Autodesk Inventor part; units mm, degrees
(part 2 of 2)
sketch "Эскиз18" plane through (0, 0, 0) normal (0, 0, -1) x (-1, 0, 0)
  line L0 (-71.0437, 196.2632) -> (-89.8727, 218.3448) projected
  arc A0 (-86.829, 224.9401) -> (-89.8727, 218.3448) centre (-86.829, 220.9401) ccw projected
  line L1 (-86.829, 224.9401) -> (-49.171, 224.9401) projected
  arc A1 (-46.1273, 218.3448) -> (-49.171, 224.9401) centre (-49.171, 220.9401) ccw projected
  line L2 (-46.1273, 218.3448) -> (-64.9563, 196.2632) projected
  arc A2 (-71.0437, 196.2632) -> (-64.9563, 196.2632) centre (-68, 198.8586) ccw projected
  line L3 (-53.9492, 66.9978) -> (-53.9492, 50.0917) projected
  arc A3 (-57.1492, 50.0917) -> (-53.9492, 50.0917) centre (-55.5492, 50.0917) ccw projected
  line L4 (-57.1492, 50.0917) -> (-57.1492, 66.9978) projected
  arc A4 (-53.9492, 66.9978) -> (-57.1492, 66.9978) centre (-55.5492, 66.9978) ccw projected
  line L5 (-23.75, 263.345) -> (-23.75, 243.345) projected
  arc A5 (-50.25, 243.345) -> (-23.75, 243.345) centre (-37, 243.345) ccw projected
  line L6 (-50.25, 243.345) -> (-50.25, 263.345) projected
  arc A6 (-23.75, 263.345) -> (-50.25, 263.345) centre (-37, 263.345) ccw projected
  line L7 (-54.45, 263.345) -> (-54.45, 243.345) projected
  arc A7 (-58.75, 243.345) -> (-54.45, 243.345) centre (-56.6, 243.345) ccw projected
  line L8 (-58.75, 243.345) -> (-58.75, 263.345) projected
  arc A8 (-54.45, 263.345) -> (-58.75, 263.345) centre (-56.6, 263.345) ccw projected
  line L9 (-19.55, 243.345) -> (-19.55, 263.345) projected
  arc A9 (-15.25, 263.345) -> (-19.55, 263.345) centre (-17.4, 263.345) ccw projected
  line L10 (-15.25, 263.345) -> (-15.25, 243.345) projected
  arc A10 (-19.55, 243.345) -> (-15.25, 243.345) centre (-17.4, 243.345) ccw projected
  line L11 (-59.5472, 66.9978) -> (-59.5472, 50.6) projected
  arc A11 (-83.5472, 50.6) -> (-59.5472, 50.6) centre (-71.5472, 50.6) ccw projected
  line L12 (-83.5472, 50.6) -> (-83.5472, 66.9978) projected
  arc A12 (-59.5472, 66.9978) -> (-83.5472, 66.9978) centre (-71.5472, 66.9978) ccw projected
  line L13 (-89.1248, 51.1083) -> (-89.1248, 58.7989) projected
  arc A13 (-89.1248, 59.3072) -> (-89.1248, 58.7989) centre (-87.5451, 59.053) ccw projected
  line L14 (-89.1248, 59.3072) -> (-89.1248, 66.9978) projected
  arc A14 (-85.9655, 66.9978) -> (-89.1248, 66.9978) centre (-87.5451, 66.9978) ccw projected
  line L15 (-85.9655, 66.9978) -> (-85.9655, 59.3072) projected
  arc A15 (-85.9655, 58.7989) -> (-85.9655, 59.3072) centre (-87.5451, 59.053) ccw projected
  line L16 (-85.9655, 58.7989) -> (-85.9655, 51.1083) projected
  arc A16 (-89.1248, 51.1083) -> (-85.9655, 51.1083) centre (-87.5451, 51.1083) ccw projected
  line L17 (-26.8046, 136.6761) -> (-52.0917, 166.3314) projected
  arc A17 (-52.0917, 172.8198) -> (-52.0917, 166.3314) centre (-48.2871, 169.5756) ccw projected
  line L18 (-52.0917, 172.8198) -> (-26.8046, 202.4751) projected
  arc A18 (-18, 199.2309) -> (-26.8046, 202.4751) centre (-23, 199.2309) ccw projected
  line L19 (-18, 199.2309) -> (-18, 139.9204) projected
  arc A19 (-26.8046, 136.6761) -> (-18, 139.9204) centre (-23, 139.9204) ccw projected
  line L20 (-109.1954, 202.4751) -> (-83.9083, 172.8198) projected
  arc A20 (-83.9083, 166.3314) -> (-83.9083, 172.8198) centre (-87.7129, 169.5756) ccw projected
  line L21 (-83.9083, 166.3314) -> (-109.1954, 136.6761) projected
  arc A21 (-118, 139.9204) -> (-109.1954, 136.6761) centre (-113, 139.9204) ccw projected
  line L22 (-118, 139.9204) -> (-118, 199.2309) projected
  arc A22 (-109.1954, 202.4751) -> (-118, 199.2309) centre (-113, 199.2309) ccw projected
  line L23 (-99.3012, 117.4553) -> (-71.8046, 149.7017) projected
  arc A23 (-64.1954, 149.7017) -> (-71.8046, 149.7017) centre (-68, 146.4575) ccw projected
  line L24 (-64.1954, 149.7017) -> (-36.6988, 117.4553) projected
  arc A24 (-40.5034, 109.2111) -> (-36.6988, 117.4553) centre (-40.5034, 114.2111) ccw projected
  line L25 (-40.5034, 109.2111) -> (-95.4966, 109.2111) projected
  arc A25 (-99.3012, 117.4553) -> (-95.4966, 109.2111) centre (-95.4966, 114.2111) ccw projected
  arc A26 (-4.2138, 22.4317) -> (0, 27.3695) centre (-5, 27.3695) ccw projected
  line L26 (0, 267.9415) -> (0, 27.3695) projected
  arc A27 (0, 267.9415) -> (-13.124, 288.8888) centre (-37, 259.345) ccw projected
  arc A28 (-13.124, 288.8888) -> (-16.2668, 290) centre (-16.2668, 285) ccw projected
  line L27 (-16.2668, 290) -> (-72.7377, 290) projected
  arc A29 (-72.7377, 290) -> (-74.4347, 289.7032) centre (-72.7377, 285) ccw projected
  arc A30 (-74.4347, 289.7032) -> (-150, 221.3595) centre (-28.8449, 163.3493) ccw projected
  line L28 (-150, 62.7066) -> (-150, 221.3595) projected
  arc A31 (-150, 62.7066) -> (-147.5924, 58.4311) centre (-145, 62.7066) ccw projected
  arc A32 (-147.1688, 58.1436) -> (-147.5924, 58.4311) centre (-150.1848, 54.1556) ccw projected
  arc A33 (-147.1688, 58.1436) -> (-4.2138, 22.4317) centre (-33.7733, 208.0855) ccw projected
  circle A34 centre (-27.8653, 29.2915) radius 2.1 projected
  circle A35 centre (-62, 278.7903) radius 2.1 projected
  circle A36 centre (-19, 278.7903) radius 2.1 projected
  circle A37 centre (-46.8597, 40.7124) radius 5.5 projected
  circle A38 centre (-8, 239.9401) radius 2.25 projected
  circle A39 centre (-8, 169.5272) radius 2.25 projected
  circle A40 centre (-8, 99.2111) radius 2.25 projected
  circle A41 centre (-81, 273) radius 5.5 projected
  circle A42 centre (-115, 59.0909) radius 5.5 projected
  circle A43 centre (-94.3579, 89.0409) radius 2.25 projected
  circle A44 centre (-142.3579, 79.1409) radius 2.25 projected
  circle A45 centre (-94.3579, 79.1409) radius 2.25 projected
  circle A46 centre (-142.3579, 89.0409) radius 2.25 projected
  line L29 (-37, 290) -> (-37, 255.5)
  circle A47 centre (-37, 255.5) radius 13.25
  circle A48 centre (-37, 239.745) radius 2.1 projected
  circle A49 centre (-37, 278.945) radius 2.1 projected
  line L30 (-37, 255.5) -> (-56.6, 255.5)
  circle A50 centre (-56.6, 255.5) radius 2.15
  circle A51 centre (-37, 235.9) radius 2.15
  circle A52 centre (-17.4, 255.5) radius 2.15
  circle A53 centre (-37, 275.1) radius 2.15
  line L31 (-71.0437, 196.2632) -> (-89.8727, 218.3448) projected
  arc A54 (-86.829, 224.9401) -> (-89.8727, 218.3448) centre (-86.829, 220.9401) ccw projected
  line L32 (-86.829, 224.9401) -> (-49.171, 224.9401) projected
  arc A55 (-46.1273, 218.3448) -> (-49.171, 224.9401) centre (-49.171, 220.9401) ccw projected
  line L33 (-46.1273, 218.3448) -> (-64.9563, 196.2632) projected
  arc A56 (-71.0437, 196.2632) -> (-64.9563, 196.2632) centre (-68, 198.8586) ccw projected
  line L34 (-53.9492, 66.9978) -> (-53.9492, 50.0917) projected
  arc A57 (-57.1492, 50.0917) -> (-53.9492, 50.0917) centre (-55.5492, 50.0917) ccw projected
  line L35 (-57.1492, 50.0917) -> (-57.1492, 66.9978) projected
  arc A58 (-53.9492, 66.9978) -> (-57.1492, 66.9978) centre (-55.5492, 66.9978) ccw projected
  line L36 (-23.75, 263.345) -> (-23.75, 243.345) projected
  arc A59 (-50.25, 243.345) -> (-23.75, 243.345) centre (-37, 243.345) ccw projected
  line L37 (-50.25, 243.345) -> (-50.25, 263.345) projected
  arc A60 (-23.75, 263.345) -> (-50.25, 263.345) centre (-37, 263.345) ccw projected
  line L38 (-54.45, 263.345) -> (-54.45, 243.345) projected
  arc A61 (-58.75, 243.345) -> (-54.45, 243.345) centre (-56.6, 243.345) ccw projected
  line L39 (-58.75, 243.345) -> (-58.75, 263.345) projected
  arc A62 (-54.45, 263.345) -> (-58.75, 263.345) centre (-56.6, 263.345) ccw projected
  line L40 (-19.55, 243.345) -> (-19.55, 263.345) projected
  arc A63 (-15.25, 263.345) -> (-19.55, 263.345) centre (-17.4, 263.345) ccw projected
  line L41 (-15.25, 263.345) -> (-15.25, 243.345) projected
  arc A64 (-19.55, 243.345) -> (-15.25, 243.345) centre (-17.4, 243.345) ccw projected
  line L42 (-59.5472, 66.9978) -> (-59.5472, 50.6) projected
  arc A65 (-83.5472, 50.6) -> (-59.5472, 50.6) centre (-71.5472, 50.6) ccw projected
  line L43 (-83.5472, 50.6) -> (-83.5472, 66.9978) projected
  arc A66 (-59.5472, 66.9978) -> (-83.5472, 66.9978) centre (-71.5472, 66.9978) ccw projected
  line L44 (-89.1248, 51.1083) -> (-89.1248, 58.7989) projected
  arc A67 (-89.1248, 59.3072) -> (-89.1248, 58.7989) centre (-87.5451, 59.053) ccw projected
  line L45 (-89.1248, 59.3072) -> (-89.1248, 66.9978) projected
  arc A68 (-85.9655, 66.9978) -> (-89.1248, 66.9978) centre (-87.5451, 66.9978) ccw projected
  line L46 (-85.9655, 66.9978) -> (-85.9655, 59.3072) projected
  arc A69 (-85.9655, 58.7989) -> (-85.9655, 59.3072) centre (-87.5451, 59.053) ccw projected
  line L47 (-85.9655, 58.7989) -> (-85.9655, 51.1083) projected
  arc A70 (-89.1248, 51.1083) -> (-85.9655, 51.1083) centre (-87.5451, 51.1083) ccw projected
  line L48 (-26.8046, 136.6761) -> (-52.0917, 166.3314) projected
  arc A71 (-52.0917, 172.8198) -> (-52.0917, 166.3314) centre (-48.2871, 169.5756) ccw projected
  line L49 (-52.0917, 172.8198) -> (-26.8046, 202.4751) projected
  arc A72 (-18, 199.2309) -> (-26.8046, 202.4751) centre (-23, 199.2309) ccw projected
  line L50 (-18, 199.2309) -> (-18, 139.9204) projected
  arc A73 (-26.8046, 136.6761) -> (-18, 139.9204) centre (-23, 139.9204) ccw projected
  line L51 (-109.1954, 202.4751) -> (-83.9083, 172.8198) projected
  arc A74 (-83.9083, 166.3314) -> (-83.9083, 172.8198) centre (-87.7129, 169.5756) ccw projected
  line L52 (-83.9083, 166.3314) -> (-109.1954, 136.6761) projected
  arc A75 (-118, 139.9204) -> (-109.1954, 136.6761) centre (-113, 139.9204) ccw projected
  line L53 (-118, 139.9204) -> (-118, 199.2309) projected
  arc A76 (-109.1954, 202.4751) -> (-118, 199.2309) centre (-113, 199.2309) ccw projected
  line L54 (-99.3012, 117.4553) -> (-71.8046, 149.7017) projected
  arc A77 (-64.1954, 149.7017) -> (-71.8046, 149.7017) centre (-68, 146.4575) ccw projected
  line L55 (-64.1954, 149.7017) -> (-36.6988, 117.4553) projected
  arc A78 (-40.5034, 109.2111) -> (-36.6988, 117.4553) centre (-40.5034, 114.2111) ccw projected
  line L56 (-40.5034, 109.2111) -> (-95.4966, 109.2111) projected
  arc A79 (-99.3012, 117.4553) -> (-95.4966, 109.2111) centre (-95.4966, 114.2111) ccw projected
  arc A80 (-4.2138, 22.4317) -> (0, 27.3695) centre (-5, 27.3695) ccw projected
  line L57 (0, 267.9415) -> (0, 27.3695) projected
  arc A81 (0, 267.9415) -> (-13.124, 288.8888) centre (-37, 259.345) ccw projected
  arc A82 (-13.124, 288.8888) -> (-16.2668, 290) centre (-16.2668, 285) ccw projected
  line L58 (-16.2668, 290) -> (-72.7377, 290) projected
  arc A83 (-72.7377, 290) -> (-74.4347, 289.7032) centre (-72.7377, 285) ccw projected
  arc A84 (-74.4347, 289.7032) -> (-150, 221.3595) centre (-28.8449, 163.3493) ccw projected
  line L59 (-150, 62.7066) -> (-150, 221.3595) projected
  arc A85 (-150, 62.7066) -> (-147.5924, 58.4311) centre (-145, 62.7066) ccw projected
  arc A86 (-147.1688, 58.1436) -> (-147.5924, 58.4311) centre (-150.1848, 54.1556) ccw projected
  arc A87 (-147.1688, 58.1436) -> (-4.2138, 22.4317) centre (-33.7733, 208.0855) ccw projected
  circle A88 centre (-27.8653, 29.2915) radius 2.1 projected
  circle A89 centre (-62, 278.7903) radius 2.1 projected
  circle A90 centre (-19, 278.7903) radius 2.1 projected
  circle A91 centre (-46.8597, 40.7124) radius 5.5 projected
  circle A92 centre (-8, 239.9401) radius 2.25 projected
  circle A93 centre (-8, 169.5272) radius 2.25 projected
  circle A94 centre (-8, 99.2111) radius 2.25 projected
  circle A95 centre (-81, 273) radius 5.5 projected
  circle A96 centre (-115, 59.0909) radius 5.5 projected
  circle A97 centre (-94.3579, 89.0409) radius 2.25 projected
  circle A98 centre (-142.3579, 79.1409) radius 2.25 projected
  circle A99 centre (-94.3579, 79.1409) radius 2.25 projected
  circle A100 centre (-142.3579, 89.0409) radius 2.25 projected
  circle A101 centre (-37, 255.5) radius 198.341
  line L60 (-71.5472, 50.6) -> (-71.5472, 66.9978)
  circle A102 centre (-71.5472, 60.1909) radius 12
  line L61 (-71.5472, 60.1909) -> (-93.4927, 60.1909)
  line L62 (-87.5451, 59.053) -> (-87.5451, 66.9978)
  circle A103 centre (-87.5451, 60.1909) radius 1.6
  circle A104 centre (-71.5472, 44.1929) radius 1.6
  circle A105 centre (-55.5492, 60.1909) radius 1.6
  circle A106 centre (-71.5472, 76.1889) radius 1.6
  line L63 (-40.5034, 229.9401) -> (-95.4966, 229.9401)
  line L64 (-99.3012, 221.6959) -> (-71.8046, 189.4495)
  line L65 (-64.1954, 189.4495) -> (-36.6988, 221.6959)
  arc A107 (-71.8046, 189.4495) -> (-64.1954, 189.4495) centre (-68, 192.6937) ccw
  arc A108 (-95.4966, 229.9401) -> (-99.3012, 221.6959) centre (-95.4966, 224.9401) ccw
  arc A109 (-36.6988, 221.6959) -> (-40.5034, 229.9401) centre (-40.5034, 224.9401) ccw
  point P0 (0, 0)
  point P1 (-15.25, 255.5)
  point P2 (-19.55, 255.5)
  point P3 (-58.75, 255.5)
  point P4 (-54.45, 255.5)
  point P5 (-35.3627, 276.4934)
  point P6 (-38.6373, 276.4934)
  point P7 (-50.25, 255.5)
  point P8 (-23.75, 255.5)
  point P9 (-53.9492, 60.1909)
  point P10 (-57.1492, 60.1909)
  point P11 (-89.1248, 60.445)
  point P12 (-85.9655, 60.445)
  point P13 (-85.9655, 59.9368)
  point P14 (-89.1248, 59.9368)
  point P15 (-59.5472, 60.1909)
  point P16 (-83.5472, 60.1909)
  point P17 (-83.2951, 62.6376)
  point P18 (-83.5472, 62.6983)
  point P19 (0, 229.9401)
  point P20 (-145.5042, 229.9401)
  point P21 (-52.0917, 166.3314)
  point P22 (-37.9053, 237.8501)
  point P23 (-36.0947, 237.8501)
  dimension "d89" = 396.682
  dimension "d84" = 34.5
  dimension "d87" = 360
  dimension "d90" = 3.2
  dimension "d93" = 360
  dimension "d99" = 5
  dimension "d100" = 5
  constraints: 16 end point, 13 centre point, 9 tangent, 8 point on circle, 8 point on line, 3 coincident, 3 vertical, 2 equal radius, 1 horizontal, 1 perpendicular, 21 other
  measures "d84" distance of L29.start L29.end
  measures "d90" diameter of A103
  measures "d99" distance between parallel lines of L32 L63
  measures "d100" radius of A107
extrude "Выдавливание16" add sketch "Эскиз18" against normal up to surface (4 mm away) contours L5 A47 L29 A53 A6 | L5 A5 L6 A47 | A47 L6 A6 A53 L29 | L7 A50 L8 A8 | L7 A7 L8 A50 | L9 A52 L10 A10 | L9 A9 L10 A52 | A34 | A37 | A48 A51 picked at (-36.9582, 240.5696)
extrude "Выдавливание17" cut sketch "Эскиз18" against normal blind 10 contours A105 | A103 L15 L61 | L61 L15 A103 | L61 L62 A103 L15 | L15 A103 L14 L61 | L61 L14 A103 L62 | A103 L61 L14 | L14 L61 A103 | A53 L29 A6 | A6 L29 A49 A53 | L29 A53 A6 | A6 A53 A49 L29 | A49 L29 A53 | A49 A53 L29 | A50 | A52 | A51 A48 | A48 A51 picked at (-36.8964, 276.9877) picked at (-37.1036, 276.9877) picked at (-37.1547, 237.7973) picked at (-36.9629, 235.0589)
extrude "Выдавливание18" cut sketch "Эскиз18" against normal blind 10 contours A109 L65 A107 L64 A108 L63
sketch "Эскиз19" plane through (0, 0, 0) normal (0, 0, -1) x (-1, 0, 0)
  arc A0 (-147.1688, 58.1436) -> (-4.2138, 22.4317) centre (-33.7733, 208.0855) ccw projected
  circle A1 centre (-27.8653, 29.2915) radius 2.1 projected
  circle A2 centre (-33.7733, 208.0855) radius 178.8917
  circle A3 centre (-10, 30.7806) radius 2.1
  circle A4 centre (-55, 30.4577) radius 2.1
  line L0 (0, 267.9415) -> (0, 27.3695) projected
  point P0 (0, 0)
  dimension "d103" = 4.2
  dimension "d104" = 4.2
  dimension "d105" = 10
  dimension "d106" = 45
  constraints: 3 centre point, 3 point on circle, 1 coincident
  measures "d103" diameter of A3
  measures "d104" diameter of A4
  measures "d105" distance from line of L0 A3.centre
  measures "d106" horizontal distance of A3.centre A4.centre
extrude "Выдавливание19" cut sketch "Эскиз19" against normal blind 10 contours A3 A2 | A2 A3 | A4 A2 | A2 A4
